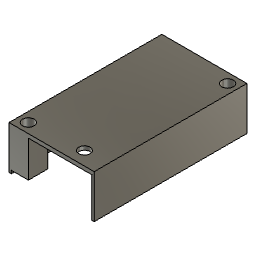
ASSEMBLAGE BOITE v2 (Autodesk Fusion 360 archive; units mm, degrees)
design "HAUT"
Autodesk Fusion 360 part; units mm, degrees
sketch "Sketch1" plane through (0, 0, 0) normal (0, 0, 1) x (1, 0, 0)
  line L0 (22, 39.5) -> (-22, 39.5)
  line L1 (-22, 39.5) -> (-22, -39.5)
  line L2 (-22, -39.5) -> (22, -39.5)
  line L3 (22, -39.5) -> (22, 39.5)
  line L4 (22, 39.5) -> (-22, -39.5) construction
  line L5 (-22, 39.5) -> (22, -39.5) construction
  dimension "d1" = 79
  dimension "d2" = 44
  constraint horizontal L0
  constraint perpendicular L0 L1
  constraint parallel L0 L2
  constraint parallel L1 L3
  constraint coincident L4 origin
  constraint coincident L5 origin
  measures "d1" distance of L0.end L1.end
  measures "d2" distance of L1.end L2.end
extrude "Extrude1" add sketch "Sketch1" along normal blind 24
shell "Shell1" thickness 1.2 removed faces 2 at (-7.3333, -39.5, 16) at (-7.3333, -13.1667, 0)
extrude "Extrude2" add 1 faces at (-7.3333, -13.1667, 24) along direction (0, 0, 1) blind 0.8
sketch "Sketch2" plane through (0, 39.5, 0) normal (0, 1, 0) x (-1, 0, 0)
  line L0 (-22, 0) -> (22, 0)
  line L1 (22, 0) -> (22, 24.8)
  line L2 (22, 24.8) -> (-22, 24.8)
  line L3 (-22, 24.8) -> (-22, 0)
  line L4 (-4.954, 16.1362) -> (-2.954, 16.1362)
  line L5 (-2.954, 16.1362) -> (-2.954, 14.1362)
  line L6 (-2.954, 14.1362) -> (-4.954, 14.1362)
  line L7 (-4.954, 14.1362) -> (-4.954, 16.1362)
  line L8 (-0.954, 16.1362) -> (1.046, 16.1362)
  line L9 (-0.954, 14.1362) -> (-0.954, 16.1362)
  line L10 (1.046, 14.1362) -> (-0.954, 14.1362)
  line L11 (1.046, 16.1362) -> (1.046, 14.1362)
  line L12 (3.046, 16.1362) -> (5.046, 16.1362)
  line L13 (3.046, 14.1362) -> (3.046, 16.1362)
  line L14 (5.046, 14.1362) -> (3.046, 14.1362)
  line L15 (5.046, 16.1362) -> (5.046, 14.1362)
  line L16 (-4.954, 12.4695) -> (-2.954, 12.4695)
  line L17 (-4.954, 10.4695) -> (-4.954, 12.4695)
  line L18 (-2.954, 10.4695) -> (-4.954, 10.4695)
  line L19 (-2.954, 12.4695) -> (-2.954, 10.4695)
  line L20 (-0.954, 12.4695) -> (1.046, 12.4695)
  line L21 (-0.954, 10.4695) -> (-0.954, 12.4695)
  line L22 (1.046, 10.4695) -> (-0.954, 10.4695)
  line L23 (1.046, 12.4695) -> (1.046, 10.4695)
  line L24 (3.046, 12.4695) -> (5.046, 12.4695)
  line L25 (3.046, 10.4695) -> (3.046, 12.4695)
  line L26 (5.046, 10.4695) -> (3.046, 10.4695)
  line L27 (5.046, 12.4695) -> (5.046, 10.4695)
  line L28 (-4.954, 8.8029) -> (-2.954, 8.8029)
  line L29 (-4.954, 6.8029) -> (-4.954, 8.8029)
  line L30 (-2.954, 6.8029) -> (-4.954, 6.8029)
  line L31 (-2.954, 8.8029) -> (-2.954, 6.8029)
  line L32 (-0.954, 8.8029) -> (1.046, 8.8029)
  line L33 (-0.954, 6.8029) -> (-0.954, 8.8029)
  line L34 (1.046, 6.8029) -> (-0.954, 6.8029)
  line L35 (1.046, 8.8029) -> (1.046, 6.8029)
  line L36 (3.046, 8.8029) -> (5.046, 8.8029)
  line L37 (3.046, 6.8029) -> (3.046, 8.8029)
  line L38 (5.046, 6.8029) -> (3.046, 6.8029)
  line L39 (5.046, 8.8029) -> (5.046, 6.8029)
  line L40 (-4.954, 5.1362) -> (-2.954, 5.1362)
  line L41 (-4.954, 3.1362) -> (-4.954, 5.1362)
  line L42 (-2.954, 3.1362) -> (-4.954, 3.1362)
  line L43 (-2.954, 5.1362) -> (-2.954, 3.1362)
  line L44 (-0.954, 5.1362) -> (1.046, 5.1362)
  line L45 (-0.954, 3.1362) -> (-0.954, 5.1362)
  line L46 (1.046, 3.1362) -> (-0.954, 3.1362)
  line L47 (1.046, 5.1362) -> (1.046, 3.1362)
  line L48 (3.046, 5.1362) -> (5.046, 5.1362)
  line L49 (3.046, 3.1362) -> (3.046, 5.1362)
  line L50 (5.046, 3.1362) -> (3.046, 3.1362)
  line L51 (5.046, 5.1362) -> (5.046, 3.1362)
  dimension "d8" = 2
  dimension "d9" = 2
  dimension "d12" = 8
  dimension "d13" = -11
  constraint horizontal L4
  constraint vertical L5
  constraint horizontal L6
  constraint vertical L7
  measures "d8" distance of L4.end L5.end
  measures "d9" distance of L4.start L4.end
extrude "Extrude3" cut sketch "Sketch2" against normal blind 7 contours L4 L5 L6 L7 | L8 L9 L10 L11 | L12 L13 L14 L15 | L16 L17 L18 L19 | L20 L21 L22 L23 | L24 L25 L26 L27 | L28 L29 L30 L31 | L32 L33 L34 L35 | L36 L37 L38 L39 | L40 L41 L42 L43 | L44 L45 L46 L47 | L48 L49 L50 L51
sketch "Sketch3" plane through (0, 0, 24.8) normal (0, 0, 1) x (-1, 0, 0)
  line L0 (-22, 39.5) -> (-22, -39.5)
  line L1 (-22, -39.5) -> (22, -39.5)
  line L2 (22, -39.5) -> (22, 39.5)
  line L3 (22, 39.5) -> (-22, 39.5)
  circle A0 centre (-9.9722, 32.5103) radius 2.9386
extrude "Extrude4" cut sketch "Sketch3" against normal blind 5 contours A0
ref_plane "WorkPlane1" through (0, 0, 25) normal (0, 0, 1) x (1, 0, 0)
sketch "Sketch4" plane through (0, 0, 25) normal (0, 0, 1) x (1, 0, 0)
  circle A0 centre (-17, -34.5) radius 3
  line L0 (-20.8, -39.5) -> (-12, -39.5)
  line L1 (-12, -39.5) -> (-12, -29.5)
  line L2 (-12, -29.5) -> (-20.8, -29.5)
  line L3 (-20.8, -29.5) -> (-20.8, -39.5)
  line L4 (-20.8, -39.5) -> (-12, -39.5)
  line L5 (-12, -39.5) -> (-12, -37.5)
  line L6 (-12, -37.5) -> (-20.8, -37.5)
  line L7 (-20.8, -37.5) -> (-20.8, -39.5)
  line L8 (-20.8, -39.5) -> (-20, -39.5)
  line L9 (-20, -39.5) -> (-20, -29.5)
  line L10 (-20, -29.5) -> (-20.8, -29.5)
  line L11 (-20.8, -29.5) -> (-20.8, -39.5)
  line L12 (-12, -39.5) -> (-14, -39.5)
  line L13 (-14, -39.5) -> (-14, -29.5)
  line L14 (-14, -29.5) -> (-12, -29.5)
  line L15 (-12, -29.5) -> (-12, -39.5)
  line L16 (-20.8, -29.5) -> (-13.268, -29.5)
  line L17 (-13.268, -29.5) -> (-13.268, -31.5)
  line L18 (-13.268, -31.5) -> (-20.8, -31.5)
  line L19 (-20.8, -31.5) -> (-20.8, -29.5)
  dimension "d19" = 6
  dimension "d21" = 0.8
  dimension "d22" = 2
  dimension "d23" = 2
  dimension "d24" = 2
  constraint horizontal L0
  constraint vertical L1
  constraint horizontal L2
  constraint vertical L3
  constraint horizontal L4
  constraint vertical L5
  constraint horizontal L6
  constraint vertical L7
  constraint coincident L1 L5.end
  constraint tangent A0 L6
  constraint horizontal L8
  constraint vertical L9
  constraint horizontal L10
  constraint vertical L11
  constraint coincident L2 L9.end
  constraint tangent A0 L9
  constraint horizontal L12
  constraint vertical L13
  constraint horizontal L14
  constraint vertical L15
  constraint coincident L2 L13.end
  constraint tangent A0 L13
  constraint horizontal L16
  constraint vertical L17
  constraint horizontal L18
  constraint vertical L19
  constraint tangent A0 L18
  measures "d19" diameter of A0
  measures "d21" distance of L0.start L8.end
  measures "d22" distance of L0.end L12.end
  measures "d23" distance of L0.end L5.end
  measures "d24" distance of L16.end L17.end
extrude "Extrude5" add sketch "Sketch4" against normal blind 23.3 contours A0 L6 L13 | L1 L2 L6 L13 L14 L15 L17 L18 | A0 L13 L18 | L2 L9 L13 L16 L18 | A0 L9 L18 | A0 L6 L9 | L0 L4 L6 L9 L13 | L0 L1 L4 L5 L6 L12 L13 L15 | L2 L13 L14 L16 L17 L18 | L3 L6 L9 L11 L18 | L2 L3 L9 L10 L11 L16 L18 L19 | L0 L3 L4 L6 L7 L8 L9 L11
extrude "Extrude6" cut 1 faces at (-12.6667, -34.5, 25) along direction (0, 0, -1) blind 0.2
extrude "Extrude7" add 1 faces at (-16.0879, -33.9171, 22.8) along direction (0, 0, -1) blind 21
extrude "Extrude8" add 1 faces at (-16.0879, -33.9171, 1.8) along direction (0, 0, -1) blind 0.1
extrude "Extrude9" cut sketch "Sketch4" against normal blind 20 contours A0
sketch "Sketch5" plane through (0, 0, 5) normal (0, 0, 1) x (-1, 0, 0)
  circle A0 centre (17, 34.5) radius 3
  circle A1 centre (17, 34.5) radius 1.6
  dimension "d35" = 3.2
  constraint concentric A0 A1
  measures "d35" diameter of A1
extrude "Extrude10" cut sketch "Sketch5" against normal blind 6 contours A1
sketch "Sketch6" plane through (0, 0, 5) normal (0, 0, 1) x (-1, 0, 0)
  circle A0 centre (17, 34.5) radius 1.6
  circle A1 centre (17, 34.5) radius 3
  line L0 (18.6, 31.9623) -> (18.6, 37.0377)
  line L1 (15.4, 37.0377) -> (15.4, 31.9623)
  line L2 (18.6, 32.9) -> (15.4, 32.9)
  line L3 (18.6, 36.1) -> (15.4, 36.1)
  constraint coincident A1 L0.start
  constraint coincident A1 L0.end
  constraint vertical L0
  constraint coincident A1 L1.start
  constraint coincident A1 L1.end
  constraint parallel L0 L1
  constraint tangent A0 L1
  constraint tangent A0 L0
  constraint coincident L0 L2.start
  constraint coincident L1 L2.end
  constraint perpendicular L1 L2
  constraint coincident L0 L3.start
  constraint coincident L1 L3.end
  constraint perpendicular L1 L3
  constraint tangent A0 L2
  constraint tangent A0 L3
extrude "Extrude11" add sketch "Sketch6" along normal blind 0.3 contours A1 L0 L1 L3 | A1 L0 L1 L2
extrude "Extrude12" add sketch "Sketch6" along normal blind 0.6 contours A1 L0 | A1 L1
extrude "Extrude13" cut 1 faces at (-13.1333, -34.5, 1.7) along direction (0, 0, 1) blind 0.2
extrude "Extrude14" cut 1 faces at (-13.1333, -34.5, 1.9) along direction (0, 0, 1) blind 0.1
sketch "Sketch8" plane through (0, 0, 24.8) normal (0, 0, 1) x (-1, 0, 0)
  circle A0 centre (17, 34.5) radius 3
  circle A1 centre (-9.9722, 32.5103) radius 2.9386
  line L0 (22, 39.5) -> (-22, 39.5)
  line L1 (-22, 39.5) -> (-22, -39.5)
  line L2 (-22, -39.5) -> (22, -39.5)
  line L3 (22, -39.5) -> (22, 39.5)
  circle A2 centre (-17, -34.5) radius 3
  line L4 (-14, -29.4839) -> (-12, -29.4839)
  line L5 (-12, -29.4839) -> (-12, -44.4839)
  line L6 (-12, -44.4839) -> (-14, -44.4839)
  line L7 (-14, -44.4839) -> (-14, -29.4839)
  line L8 (-34, -29.5) -> (-14, -29.5)
  line L9 (-14, -29.5) -> (-14, -31.5)
  line L10 (-14, -31.5) -> (-34, -31.5)
  line L11 (-34, -31.5) -> (-34, -29.5)
  line L12 (-22, -39.5) -> (-12, -39.5)
  line L13 (-12, -39.5) -> (-12, -29.4839)
  line L14 (-12, -29.4839) -> (-22, -29.4839)
  line L15 (-22, -29.4839) -> (-22, -39.5)
  dimension "d49" = 6
  dimension "d50" = 2
  dimension "d51" = 2
  dimension "d52" = 15
  dimension "d53" = 20
  constraint horizontal L4
  constraint vertical L5
  constraint horizontal L6
  constraint vertical L7
  constraint horizontal L8
  constraint vertical L9
  constraint horizontal L10
  constraint vertical L11
  constraint coincident L7 L9.end
  constraint tangent A2 L10
  constraint tangent A2 L7
  constraint horizontal L12
  constraint vertical L13
  constraint horizontal L14
  constraint vertical L15
  constraint coincident L1.end L2.start
  measures "d49" diameter of A2
  measures "d50" distance of L8.end L9.end
  measures "d51" distance of L4.start L4.end
  measures "d52" distance of L4.end L5.end
  measures "d53" distance of L8.start L8.end
extrude "Extrude15" add sketch "Sketch8" against normal blind 23 contours L2 L4 L5 L7 L9 L12 L13 L14 | L1 L7 L8 L9 L10 L15 | L1 L2 A2 L7 L10 L12 L15 | A2 | A2 L7 L10
extrude "Extrude16" cut sketch "Sketch8" against normal blind 19.2 contours A2
sketch "Sketch9" plane through (0, 0, 5.6) normal (0, 0, 1) x (-1, 0, 0)
  circle A0 centre (-17, -34.5) radius 3
  circle A1 centre (-17, -34.5) radius 1.6
  dimension "d58" = 3.2
  constraint concentric A0 A1
  measures "d58" diameter of A1
extrude "Extrude17" cut sketch "Sketch9" against normal blind 13 contours A1
sketch "Sketch10" plane through (0, 0, 5.6) normal (0, 0, 1) x (-1, 0, 0)
  circle A0 centre (-17, -34.5) radius 1.6
  circle A1 centre (-17, -34.5) radius 3
  line L0 (-15.4738, -37.0828) -> (-15.3275, -32.0094)
  line L1 (-18.6, -31.9623) -> (-18.6, -37.0377)
  line L2 (-15.4455, -36.1) -> (-18.6, -36.1)
  line L3 (-18.6, -32.9) -> (-15.3532, -32.9)
  constraint coincident A1 L0.start
  constraint coincident A1 L0.end
  constraint coincident A1 L1.start
  constraint coincident A1 L1.end
  constraint vertical L1
  constraint tangent A0 L1
  constraint tangent A0 L0
  constraint coincident L0 L2.start
  constraint coincident L1 L2.end
  constraint perpendicular L1 L2
  constraint coincident L1 L3.start
  constraint coincident L0 L3.end
  constraint perpendicular L1 L3
  constraint tangent A0 L2
  constraint tangent A0 L3
extrude "Extrude18" cut sketch "Sketch10" against normal blind 0.3 contours A1 L0 L1 L3 | A1 L0 L1 L2
extrude "Extrude19" cut sketch "Sketch10" against normal blind 0.6 contours A0 L0 L2 | A0 L0 L3 | A0 L1 L3 | A0 L1 L2
extrude "Extrude20" add 1 faces at (-6.9333, 12.7613, 22.8) along direction (0, 0, -1) blind 2
extrude "Extrude21" cut 1 faces at (-7.7343, 13.3598, 24.8) along direction (0, 0, -1) blind 2
sketch "Sketch12" plane through (0, 0, 20.8) normal (0, 0, -1) x (1, 0, 0)
  line L0 (14, -29.5) -> (20.8, -29.5)
  line L1 (20.8, -29.5) -> (20.8, 39.5)
  line L2 (20.8, 39.5) -> (-12, 39.5)
  line L3 (-12, 39.5) -> (-12, 29.5)
  line L4 (-12, 29.5) -> (-20.8, 29.5)
  line L5 (-20.8, 29.5) -> (-20.8, -38.3)
  line L6 (-20.8, -38.3) -> (12, -38.3)
  line L7 (12, -38.3) -> (12, -29.4839)
  line L8 (12, -29.4839) -> (14, -29.4839)
  line L9 (14, -29.4839) -> (14, -29.5)
  circle A0 centre (9.9722, 32.5103) radius 2.9386
  line L10 (-14.8733, 29.3964) -> (-14.8733, -35.7877) construction
  line L11 (-14.8733, -35.7877) -> (4.8049, -35.7877) construction
  line L12 (4.8049, -35.7877) -> (4.8049, 29.3964) construction
  line L13 (4.8049, 29.3964) -> (-14.8733, 29.3964) construction
  dimension "d74" = 8
  text T0 "TD2 - Gr05" font "Arial Black" height 8 align left top in box 65.1841 x 19.6782 at (-14.8733, 29.3964) x (0, -1) y (1, 0) spacing 1 kerned
extrude "Extrude23" cut sketch "Sketch12" against normal blind 0.5 text T0
extrude "Extrude24" cut 1 faces at (-21.6, 12.7667, 0) along direction (0, 0, 1) blind 0.4
equation "d22 = 0.8 mm + 1.2 mm"
